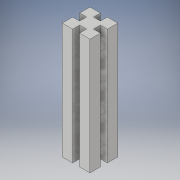
# Autodesk Inventor part: Maze Wall Post
Saved by Autodesk Inventor 2019 (Build 230136000, 136)
## iProperties
Created: 2019-01-24
Part Number: Maze Wall Post
Material: Generic
Document SubType Name: Modeling
Designer: Billy
Density: 1 g/cm^3
Appearance: Default
Author: Billy
Autodesk Inventor part; units mm, degrees
ref_plane "YZ Plane" through (0, 0, 0) normal (1, 0, 0) x (0, 1, 0)
ref_plane "XZ Plane" through (0, 0, 0) normal (0, 1, 0) x (-1, 0, 0)
sketch "Sketch1" plane through (0, 0, 0) normal (0, 1, 0) x (-1, 0, 0)
  line L0 (0, -8.85) -> (0, -7.5)
  line L1 (0, -4.5) -> (0, -3.15)
  line L2 (3, -6) -> (3, -7.5)
  line L3 (3, -7.5) -> (0, -7.5)
  line L4 (0, -4.5) -> (3, -4.5)
  line L5 (3, -4.5) -> (3, -6)
  line L6 (4.5, -12) -> (4.5, -9)
  line L7 (4.5, -9) -> (6, -9)
  line L8 (6, -9) -> (7.5, -9)
  line L9 (7.5, -9) -> (7.5, -12)
  line L10 (12, -7.5) -> (9, -7.5)
  line L11 (9, -7.5) -> (9, -6)
  line L12 (9, -6) -> (9, -4.5)
  line L13 (9, -4.5) -> (12, -4.5)
  line L14 (7.5, 0) -> (7.5, -3)
  line L15 (7.5, -3) -> (6, -3)
  line L16 (6, -3) -> (4.5, -3)
  line L17 (4.5, -3) -> (4.5, 0)
  line L18 (12, 0) -> (12, -4.5)
  line L19 (12, -7.5) -> (12, -12)
  line L20 (12, -12) -> (7.5, -12)
  line L21 (4.5, -12) -> (0, -12)
  line L22 (0, 0) -> (4.5, 0)
  line L23 (7.5, 0) -> (12, 0)
  line L24 (0, -12) -> (0, -7.5)
  line L25 (0, -4.5) -> (0, 0)
  point P0 (6, -6)
  dimension "d10" = 360
  dimension "d1" = 12
  constraints: 52 end point, 8 parallel, 4 perpendicular, 2 horizontal, 1 point on line, 37 other
  measures "d1" distance of L18.start L19.end
extrude "Extrusion1" add sketch "Sketch1" along normal blind 50
ref_plane "Work Plane1" through (0, 3, 0) normal (0, -1, 0) x (1, 0, 0)
sketch "Sketch6" plane through (0, 3, 0) normal (0, -1, 0) x (1, 0, 0)
  line L0 (-8.6812, -4.452) -> (-7.3406, -3.678) projected
  line L1 (-7.3406, -3.678) -> (-6.1663, -3) projected
  line L2 (-6.1663, -3) -> (-5.8337, -3) projected
  line L3 (-5.8337, -3) -> (-4.6594, -3.678) projected
  line L4 (-4.6594, -3.678) -> (-3.3187, -4.452) projected
  line L5 (-3.3187, -4.452) -> (-3.3188, -6) projected
  line L6 (-3.3188, -6) -> (-3.3188, -12) projected
  line L7 (-3.3188, -12) -> (-4.5, -12) projected
  line L8 (-4.5, -12) -> (-4.5, -9) projected
  line L9 (-4.5, -9) -> (-7.5, -9) projected
  line L10 (-7.5, -9) -> (-7.5, -12) projected
  line L11 (-7.5, -12) -> (-8.6812, -12) projected
  line L12 (-8.6812, -12) -> (-8.6812, -6) projected
  line L13 (-8.6812, -6) -> (-8.6812, -4.452) projected
  point P0 (0, 0)
extrude "Extrusion2" cut sketch "Sketch6" against normal blind 4
sketch "Sketch7" plane through (0, 0, 0) normal (0, -1, 0) x (1, 0, 0)
  line L0 (0, 0) -> (0, -4.5) projected
  line L1 (-4.5, 0) -> (0, 0) projected
  line L2 (-4.5, -3) -> (-4.5, 0) projected
  line L3 (-7.5, -3) -> (-4.5, -3) projected
  line L4 (-7.5, 0) -> (-7.5, -3) projected
  line L5 (-12, 0) -> (-7.5, 0) projected
  line L6 (-12, -4.5) -> (-12, 0) projected
  line L7 (-9, -4.5) -> (-12, -4.5) projected
  line L8 (-9, -7.5) -> (-9, -4.5) projected
  line L9 (-12, -7.5) -> (-9, -7.5) projected
  line L10 (-12, -12) -> (-12, -7.5) projected
  line L11 (-7.5, -12) -> (-12, -12) projected
  line L12 (-7.5, -9) -> (-7.5, -12) projected
  line L13 (-4.5, -9) -> (-7.5, -9) projected
  line L14 (-4.5, -12) -> (-4.5, -9) projected
  line L15 (0, -12) -> (-4.5, -12) projected
  line L16 (0, -7.5) -> (0, -12) projected
  line L17 (-3, -7.5) -> (0, -7.5) projected
  line L18 (-3, -4.5) -> (-3, -7.5) projected
  line L19 (0, -4.5) -> (-3, -4.5) projected
  circle A0 centre (-6, -6) radius 1.6
  dimension "d26" = 3.2
  constraints: 1 centre point
  measures "d26" diameter of A0
extrude "Extrusion3" cut sketch "Sketch7" against normal blind 25.4 contours A0
sketch "Sketch8" plane through (-7.5, 0, -12) normal (0, 0, -1) x (-1, 0, 0)
  line L0 (-3, 7) -> (0, 7)
  line L1 (-3, 50) -> (0, 50)
  line L2 (-1.6663, 3) -> (-4.1813, 3)
  line L3 (-1.6663, 7) -> (-4.1813, 7)
  line L4 (-4.1813, 3) -> (-4.1813, 7)
  line L5 (0, 3) -> (-3, 3)
  line L6 (-3, 0) -> (0, 0)
  line L7 (1.1812, 3) -> (-0.1594, 3)
  line L8 (1.1812, 3) -> (1.1812, 7)
  line L9 (1.1812, 7) -> (-0.1594, 7)
  point P0 (-7.5, 0)
  constraints: 20 end point, 8 point on line
extrude "Extrusion4" cut sketch "Sketch8" against normal up to surface (9 mm away)
body "Solid1"
